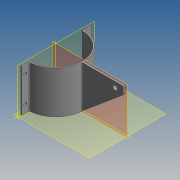
# Autodesk Inventor part: P050_SupportTube2
Saved by Autodesk Inventor 2021.3 (Build 253353000, 353)
## iProperties
Created: 2022-01-14
Part Number: P050_SupportTube2
Material: Générique
Document SubType Name: Modeling
Designer: gabri
Density: 1 g/cm^3
Appearance: Par défaut
Author: gabri
Autodesk Inventor part; units mm, degrees
sketch "Sketch2" plane through (0, 0, 0) normal (0, 0, 1) x (1, 0, 0)
  arc A0 (0, -52) -> (0, 52) centre (0, 0) ccw
  arc A1 (0, -50) -> (0, 50) centre (0, 0) ccw
  line L0 (0, 52) -> (0, 50)
  line L1 (0, -50) -> (0, -52)
  line L2 (0, -50) -> (2, -50)
  line L3 (2, -50) -> (2, -66)
  line L4 (2, -66) -> (0, -66)
  line L5 (0, -66) -> (0, -50)
  line L6 (0, 50) -> (2, 50)
  line L7 (2, 50) -> (2, 66)
  line L8 (2, 66) -> (0, 66)
  line L9 (0, 66) -> (0, 50)
  point P0 (0, 52)
  point P1 (2, 51.9615)
  point P2 (2, -51.9615)
  dimension "d0" = 104
  dimension "d1" = 100
  dimension "d2" = 2
  dimension "d5" = 2
  dimension "d6" = 16
  dimension "d7" = 2
  dimension "d8" = 16
  constraints: 20 end point, 4 parallel, 4 point on circle, 2 centre point, 2 coincident, 2 horizontal, 2 perpendicular, 2 point on line, 1 vertical
  measures "d0" diameter of A0
  measures "d1" diameter of A1
  measures "d2" distance of L0.start L0.end
  measures "d5" distance between parallel lines of L3 L5
  measures "d6" distance from line of L2 L4.end
  measures "d7" distance between parallel lines of L7 L9
  measures "d8" distance between parallel lines of L6 L8
extrude "Extrusion1" add sketch "Sketch2" along normal blind 80
fillet "Fillet1" radius 2 2 edges at (2, -51.9615, 40) (2, 51.9615, 40)
sketch "Sketch3" plane through (2, -66, 80) normal (1, 0, 0) x (0, 0, -1)
  line L0 (80, 16) -> (80, 0) construction
  line L1 (80, 0) -> (0, 0) construction
  line L2 (0, 16) -> (0, 0) construction
  line L3 (80, 16) -> (0, 16) construction
  line L4 (80, 132) -> (80, 116) construction
  line L5 (80, 116) -> (0, 116) construction
  line L6 (0, 132) -> (0, 116) construction
  line L7 (80, 132) -> (0, 132) construction
  point P0 (80, 66)
  point P1 (15, 6)
  point P2 (65, 6)
  point P3 (15, 126)
  point P4 (65, 126)
  dimension "d10" = 15
  dimension "d11" = 15
  dimension "d12" = 15
  dimension "d13" = 15
  dimension "d14" = 6
  dimension "d15" = 6
  dimension "d16" = 6
  dimension "d17" = 6
  measures "d10" distance from line of point (15, 6) L2
  measures "d11" distance from line of L6 point (15, 126)
  measures "d12" distance from line of point (65, 6) L0
  measures "d13" distance from line of point (65, 126) L4
  measures "d14" distance from line of point (65, 6) L1
  measures "d15" distance from line of L1 point (15, 6)
  measures "d16" distance from line of L7 point (15, 126)
  measures "d17" distance from line of L7 point (65, 126)
hole "Hole1" at (2, -60, 65) at (2, -60, 15) at (2, 60, 65) at (2, 60, 15) direction (-1, 0, 0) diameter 6.5 depth 2 tip angle 118
sketch "Sketch4" plane through (0, 0, 0) normal (0, 1, 0) x (-1, 0, 0)
  line L0 (-3.8519, 80) -> (-3.8519, 0) construction
  line L1 (-3.8519, 80) -> (-3.8519, 80) construction
  line L2 (-3.8519, 0) -> (-3.8519, 80) construction
  line L3 (-3.8519, 0) -> (-3.8519, 0) construction
  line L4 (-52, 0) -> (-52, 80) construction
  line L5 (-50, 80) -> (-130, 80)
  line L6 (-130, 80) -> (-130, 65.4498)
  line L7 (-130, 65.4498) -> (-52, 0)
  line L8 (-52, 0) -> (-49.7983, 0)
  line L9 (-50, 80) -> (-50, 0) construction
  line L10 (-52, 0) -> (-50, 0)
  line L11 (-50, 0) -> (-50, 80)
  line L12 (-50, 80) -> (-50, 80)
  point P0 (0, 0)
  dimension "d25" = 80
  dimension "d26" = 130
  constraints: 14 end point, 2 collinear, 2 horizontal, 2 perpendicular, 1 midpoint
  measures "d25" distance of L5.start L5.end
  measures "d26" angle of L7 L6
extrude "Extrusion2" add sketch "Sketch4" along normal mid plane 4
sketch "Sketch5" plane through (0, -2, 0) normal (0, -1, 0) x (1, 0, 0)
  line L0 (130, 80) -> (51.9615, 80) construction
  line L1 (130, 65.4498) -> (130, 80) construction
  point P0 (0, 0)
  point P1 (115, 70)
  point P2 (52, 80)
  dimension "d29" = 10
  dimension "d30" = 15
  measures "d29" distance from line of point (115, 70) L0
  measures "d30" distance from line of L1 point (115, 70)
hole "Hole2" at (115, -2, 70) direction (0, 1, 0) diameter 8.5 depth 4 tip angle 118
fillet "Fillet2" radius 2 2 edges at (130, 0, 80) (130, 0, 65.4498)
fillet "Fillet3" radius 2 2 edges at (51.9615, -2, 40) (51.9615, 2, 40)
body "Solid1"
